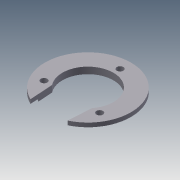
# Autodesk Inventor part: DispenserHolderCapturePlate
Saved by Autodesk Inventor 2012 SP1 (Build 160190100, 190)
## iProperties
Created: 2010-02-11
Part Number: DispenserHolderCapturePlate
Document SubType Name: Modeling
Designer: rconnaug
Density: 2.71 g/cm^3
Material: Aluminum-6061
Mass: 2.77703 g
Surface Area: 13.4064 cm^2
Volume: 1.02473 cm^3
Author: rconnaug
Autodesk Inventor part; units mm, degrees
ref_plane "YZ Plane" through (0, 0, 0) normal (1, 0, 0) x (0, 1, 0)
ref_plane "XZ Plane" through (0, 0, 0) normal (0, 1, 0) x (-1, 0, 0)
ref_plane "XY Plane" through (0, 0, 0) normal (0, 0, 1) x (1, 0, 0)
sketch "Sketch2" plane through (0, 0, 0) normal (0, 1, 0) x (-1, 0, 0)
  arc A0 (-7.5, 15.7699) -> (7.5, 15.7699) centre (0, 0) ccw
  arc A1 (-8.128, 6.3879) -> (8.128, 6.3879) centre (0, 0) ccw
  line L0 (7.5, 15.7699) -> (8.128, 6.3879)
  line L1 (-8.128, 6.3879) -> (-7.5, 15.7699)
  line L2 (8.128, 6.3879) -> (-8.128, 6.3879) construction
  line L3 (-7.5, 15.7699) -> (7.5, 15.7699) construction
  dimension "d0" = 34.925
  dimension "d1" = 20.6756
  dimension "d2" = 16.256
  dimension "d3" = 15
  constraints: 8 end point, 4 point on circle, 2 centre point, 2 coincident, 1 horizontal, 1 parallel
  measures "d0" diameter of A0
  measures "d1" diameter of A1
  measures "d2" distance of L1.start L0.end
  measures "d3" distance of L1.end L0.start
extrude "Extrusion1" add sketch "Sketch2" along normal blind 1.65
sketch "Sketch3" plane through (0, 0, 0) normal (0, -1, 0) x (1, 0, 0)
  line L0 (7.5, 15.7699) -> (8.128, 6.3879) projected
  arc A0 (-8.128, 6.3879) -> (8.128, 6.3879) centre (0, 0) ccw projected
  line L1 (-8.128, 6.3879) -> (-7.5, 15.7699) projected
  arc A1 (-7.726, 12.3942) -> (7.726, 12.3942) centre (0, 0) ccw
  arc A2 (-8.128, 6.3879) -> (8.128, 6.3879) centre (0, 0) ccw
  line L2 (-8.128, 6.3879) -> (-7.726, 12.3942)
  line L3 (8.128, 6.3879) -> (7.726, 12.3942)
  dimension "d6" = 29.21
  constraints: 4 end point, 4 point on circle, 2 centre point, 2 coincident, 2 point on line, 1 concentric
  measures "d6" diameter of A1
extrude "Extrusion2" add sketch "Sketch3" along normal blind 1
sketch "Sketch4" plane through (0, 1.65, 0) normal (0, 1, 0) x (1, 0, 0)
  arc A0 (7.5, -15.7699) -> (-7.5, -15.7699) centre (0, 0) ccw projected
  line L0 (0, 24.109) -> (0, -22.4163) projected
  point P0 (0, 13.0302)
  dimension "d9" = 13.0302
  constraints: 1 point on line
  measures "d9" distance of A0.centre point (0, 13.03)
hole "Hole1" at (0, 1.65, -13.0302) direction (0, -1, 0) diameter 2.6416 end through all clearance for "Flat Head Machine Screw (82)" size "#3" standard "Ansi Unified Screw Threads"
pattern_circular "Circular Pattern1" count 3 over 360 about axis through (0, 0, 0) along (0, 1, 0) of "Hole1"
body "Solid1"
